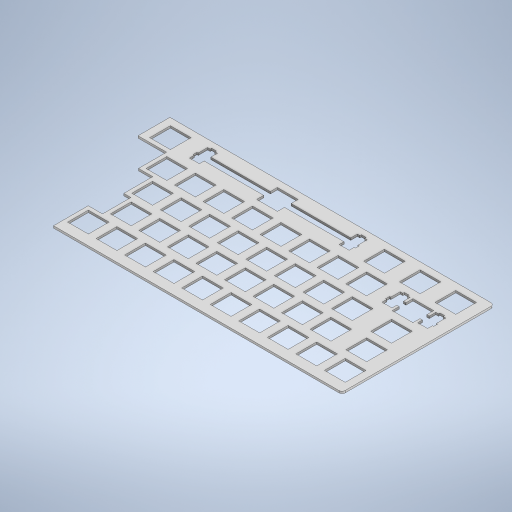
# Autodesk Inventor part: case_plate_p1
Saved by Autodesk Inventor 2024 (Build 280153000, 153)
## iProperties
Created: 2023-08-02
Part Number: case_plate_p1
Material: Generic
Document SubType Name: Modeling
Designer: Mika
Density: 1 g/cm^3
Appearance: Default
Author: Mika
Autodesk Inventor part; units mm, degrees
ref_plane "YZ Plane" through (0, 0, 0) normal (1, 0, 0) x (0, 1, 0)
ref_plane "XZ Plane" through (0, 0, 0) normal (0, 1, 0) x (-1, 0, 0)
ref_plane "XY Plane" through (0, 0, 0) normal (0, 0, 1) x (1, 0, 0)
sketch "Sketch1" plane through (0, 0, 0) normal (0, 1, 0) x (-1, 0, 0)
  line L0 (309.0479, 99.8402) -> (309.0479, 2.3404)
  line L1 (307.045, 0.3402) -> (2.0931, 0.3389)
  line L2 (0.096, 2.3404) -> (0.096, 99.8389)
  line L3 (2.096, 101.8389) -> (307.045, 101.8402)
  line L4 (126.213, 18.8654) -> (126.213, 14.1663)
  line L5 (126.213, 14.1663) -> (86.4387, 14.1663)
  line L6 (86.4387, 14.1663) -> (86.4387, 17.395)
  line L7 (86.4387, 17.395) -> (84.7136, 17.395)
  line L8 (81.5633, 17.395) -> (79.8382, 17.395)
  line L9 (79.8382, 17.395) -> (79.8382, 14.1663)
  line L10 (79.8382, 14.1663) -> (79.0141, 14.1663)
  line L11 (79.0141, 14.1663) -> (79.0141, 11.5163)
  line L12 (79.0141, 11.5163) -> (79.8382, 11.5163)
  line L13 (79.8382, 11.5163) -> (79.8382, 5.2462)
  line L14 (79.8382, 5.2462) -> (81.5633, 5.2462)
  line L15 (81.5633, 5.2462) -> (81.5633, 4.265)
  line L16 (81.5633, 4.265) -> (84.7136, 4.265)
  line L17 (84.7136, 4.265) -> (84.7136, 5.2462)
  line L18 (84.7136, 5.2462) -> (86.4387, 5.2462)
  line L19 (86.4387, 5.2462) -> (86.4387, 9.7166)
  line L20 (86.4387, 9.7166) -> (126.213, 9.7166)
  line L21 (126.213, 9.7166) -> (126.213, 5.0161)
  line L22 (126.213, 5.0161) -> (140.064, 5.0161)
  line L23 (140.064, 5.0161) -> (140.064, 9.7166)
  line L24 (140.064, 9.7166) -> (179.838, 9.7166)
  line L25 (179.838, 9.7166) -> (179.838, 5.2462)
  line L26 (179.838, 5.2462) -> (181.563, 5.2462)
  line L27 (181.563, 5.2462) -> (181.563, 4.265)
  line L28 (181.563, 4.265) -> (184.714, 4.265)
  line L29 (184.714, 4.265) -> (184.714, 5.2462)
  line L30 (184.714, 5.2462) -> (186.439, 5.2462)
  line L31 (186.439, 5.2462) -> (186.439, 11.5163)
  line L32 (186.439, 11.5163) -> (187.263, 11.5163)
  line L33 (187.263, 11.5163) -> (187.263, 14.1663)
  line L34 (187.263, 14.1663) -> (186.439, 14.1663)
  line L35 (186.439, 14.1663) -> (186.439, 17.395)
  line L36 (186.439, 17.395) -> (184.714, 17.395)
  line L37 (181.563, 17.395) -> (179.838, 17.395)
  line L38 (179.838, 17.395) -> (179.838, 14.1663)
  line L39 (179.838, 14.1663) -> (140.064, 14.1663)
  line L40 (140.064, 14.1663) -> (140.064, 18.8654)
  line L41 (140.064, 18.8654) -> (126.213, 18.8654)
  line L42 (7.152, 18.8654) -> (21.0013, 18.8654)
  line L43 (21.0013, 18.8654) -> (21.0013, 5.0161)
  line L44 (21.0013, 5.0161) -> (7.152, 5.0161)
  line L45 (7.152, 5.0161) -> (7.152, 18.8654)
  line L46 (30.9631, 18.8654) -> (44.8137, 18.8654)
  line L47 (44.8137, 18.8654) -> (44.8137, 5.0161)
  line L48 (44.8137, 5.0161) -> (30.9631, 5.0161)
  line L49 (30.9631, 5.0161) -> (30.9631, 18.8654)
  line L50 (54.7769, 18.8654) -> (68.6262, 18.8654)
  line L51 (68.6262, 18.8654) -> (68.6262, 5.0161)
  line L52 (68.6262, 5.0161) -> (54.7769, 5.0161)
  line L53 (54.7769, 5.0161) -> (54.7769, 18.8654)
  line L54 (197.652, 18.8654) -> (211.501, 18.8654)
  line L55 (211.501, 18.8654) -> (211.501, 5.0161)
  line L56 (211.501, 5.0161) -> (197.652, 5.0161)
  line L57 (197.652, 5.0161) -> (197.652, 18.8654)
  line L58 (221.463, 18.8654) -> (235.314, 18.8654)
  line L59 (235.314, 18.8654) -> (235.314, 5.0161)
  line L60 (235.314, 5.0161) -> (221.463, 5.0161)
  line L61 (221.463, 5.0161) -> (221.463, 18.8654)
  line L62 (252.421, 18.8654) -> (266.27, 18.8654)
  line L63 (266.27, 18.8654) -> (266.27, 5.0161)
  line L64 (266.27, 5.0161) -> (252.421, 5.0161)
  line L65 (252.421, 5.0161) -> (252.421, 18.8654)
  line L66 (271.471, 18.8654) -> (285.32, 18.8654)
  line L67 (285.32, 18.8654) -> (285.32, 5.0161)
  line L68 (285.32, 5.0161) -> (271.471, 5.0161)
  line L69 (271.471, 5.0161) -> (271.471, 18.8654)
  line L70 (290.521, 18.8654) -> (304.37, 18.8654)
  line L71 (304.37, 18.8654) -> (304.37, 5.0161)
  line L72 (304.37, 5.0161) -> (290.521, 5.0161)
  line L73 (290.521, 5.0161) -> (290.521, 18.8654)
  line L74 (16.677, 37.9155) -> (16.677, 33.2163)
  line L75 (16.677, 33.2163) -> (15.0013, 33.2163)
  line L76 (15.0013, 33.2163) -> (15.0013, 36.4451)
  line L77 (15.0013, 36.4451) -> (13.276, 36.4451)
  line L78 (10.1258, 36.4451) -> (8.4019, 36.4451)
  line L79 (8.4019, 36.4451) -> (8.4019, 33.2163)
  line L80 (8.4019, 33.2163) -> (7.5765, 33.2163)
  line L81 (7.5765, 33.2163) -> (7.5765, 30.5663)
  line L82 (7.5765, 30.5663) -> (8.4019, 30.5663)
  line L83 (8.4019, 30.5663) -> (8.4019, 24.2962)
  line L84 (8.4019, 24.2962) -> (10.1258, 24.2962)
  line L85 (10.1258, 24.2962) -> (10.1258, 23.315)
  line L86 (10.1258, 23.315) -> (13.276, 23.315)
  line L87 (13.276, 23.315) -> (13.276, 24.2962)
  line L88 (13.276, 24.2962) -> (15.0013, 24.2962)
  line L89 (15.0013, 24.2962) -> (15.0013, 28.7652)
  line L90 (15.0013, 28.7652) -> (16.677, 28.7652)
  line L91 (16.677, 28.7652) -> (16.677, 24.0661)
  line L92 (16.677, 24.0661) -> (30.5263, 24.0661)
  line L93 (30.5263, 24.0661) -> (30.5263, 28.7652)
  line L94 (30.5263, 28.7652) -> (32.202, 28.7652)
  line L95 (32.202, 28.7652) -> (32.202, 24.2962)
  line L96 (32.202, 24.2962) -> (33.9259, 24.2962)
  line L97 (33.9259, 24.2962) -> (33.9259, 23.315)
  line L98 (33.9259, 23.315) -> (37.0762, 23.315)
  line L99 (37.0762, 23.315) -> (37.0762, 24.2962)
  line L100 (37.0762, 24.2962) -> (38.8013, 24.2962)
  line L101 (38.8013, 24.2962) -> (38.8013, 30.5663)
  line L102 (38.8013, 30.5663) -> (39.6268, 30.5663)
  line L103 (39.6268, 30.5663) -> (39.6268, 33.2163)
  line L104 (39.6268, 33.2163) -> (38.8013, 33.2163)
  line L105 (38.8013, 33.2163) -> (38.8013, 36.4451)
  line L106 (38.8013, 36.4451) -> (37.0762, 36.4451)
  line L107 (33.9259, 36.4451) -> (32.202, 36.4451)
  line L108 (32.202, 36.4451) -> (32.202, 33.2163)
  line L109 (32.202, 33.2163) -> (30.5263, 33.2163)
  line L110 (30.5263, 33.2163) -> (30.5263, 37.9155)
  line L111 (30.5263, 37.9155) -> (16.677, 37.9155)
  line L112 (47.6321, 37.9155) -> (61.4825, 37.9155)
  line L113 (61.4825, 37.9155) -> (61.4825, 24.0661)
  line L114 (61.4825, 24.0661) -> (47.6321, 24.0661)
  line L115 (47.6321, 24.0661) -> (47.6321, 37.9155)
  line L116 (66.6821, 37.9155) -> (80.5325, 37.9155)
  line L117 (80.5325, 37.9155) -> (80.5325, 24.0661)
  line L118 (80.5325, 24.0661) -> (66.6821, 24.0661)
  line L119 (66.6821, 24.0661) -> (66.6821, 37.9155)
  line L120 (85.7321, 37.9155) -> (99.5825, 37.9155)
  line L121 (99.5825, 37.9155) -> (99.5825, 24.0661)
  line L122 (99.5825, 24.0661) -> (85.7321, 24.0661)
  line L123 (85.7321, 24.0661) -> (85.7321, 37.9155)
  line L124 (104.782, 37.9155) -> (118.632, 37.9155)
  line L125 (118.632, 37.9155) -> (118.632, 24.0661)
  line L126 (118.632, 24.0661) -> (104.782, 24.0661)
  line L127 (104.782, 24.0661) -> (104.782, 37.9155)
  line L128 (123.832, 37.9155) -> (137.682, 37.9155)
  line L129 (137.682, 37.9155) -> (137.682, 24.0661)
  line L130 (137.682, 24.0661) -> (123.832, 24.0661)
  line L131 (123.832, 24.0661) -> (123.832, 37.9155)
  line L132 (142.882, 37.9155) -> (156.732, 37.9155)
  line L133 (156.732, 37.9155) -> (156.732, 24.0661)
  line L134 (156.732, 24.0661) -> (142.882, 24.0661)
  line L135 (142.882, 24.0661) -> (142.882, 37.9155)
  line L136 (161.932, 37.9155) -> (175.782, 37.9155)
  line L137 (175.782, 37.9155) -> (175.782, 24.0661)
  line L138 (175.782, 24.0661) -> (161.932, 24.0661)
  line L139 (161.932, 24.0661) -> (161.932, 37.9155)
  line L140 (180.982, 37.9155) -> (194.832, 37.9155)
  line L141 (194.832, 37.9155) -> (194.832, 24.0661)
  line L142 (194.832, 24.0661) -> (180.982, 24.0661)
  line L143 (180.982, 24.0661) -> (180.982, 37.9155)
  line L144 (200.032, 37.9155) -> (213.882, 37.9155)
  line L145 (213.882, 37.9155) -> (213.882, 24.0661)
  line L146 (213.882, 24.0661) -> (200.032, 24.0661)
  line L147 (200.032, 24.0661) -> (200.032, 37.9155)
  line L148 (219.082, 37.9155) -> (232.932, 37.9155)
  line L149 (232.932, 37.9155) -> (232.932, 24.0661)
  line L150 (232.932, 24.0661) -> (219.082, 24.0661)
  line L151 (219.082, 24.0661) -> (219.082, 37.9155)
  line L152 (245.277, 37.9155) -> (259.126, 37.9155)
  line L153 (259.126, 37.9155) -> (259.126, 24.0661)
  line L154 (259.126, 24.0661) -> (245.277, 24.0661)
  line L155 (245.277, 24.0661) -> (245.277, 37.9155)
  line L156 (271.471, 37.9155) -> (285.32, 37.9155)
  line L157 (285.32, 37.9155) -> (285.32, 24.0661)
  line L158 (285.32, 24.0661) -> (271.471, 24.0661)
  line L159 (271.471, 24.0661) -> (271.471, 37.9155)
  line L160 (290.521, 37.9155) -> (304.37, 37.9155)
  line L161 (304.37, 37.9155) -> (304.37, 24.0661)
  line L162 (304.37, 24.0661) -> (290.521, 24.0661)
  line L163 (290.521, 24.0661) -> (290.521, 37.9155)
  line L164 (259.563, 56.9655) -> (259.563, 52.2661)
  line L165 (259.563, 52.2661) -> (257.889, 52.2661)
  line L166 (257.889, 52.2661) -> (257.889, 55.4951)
  line L167 (257.889, 55.4951) -> (256.162, 55.4951)
  line L168 (253.013, 55.4951) -> (251.288, 55.4951)
  line L169 (251.288, 55.4951) -> (251.288, 52.2661)
  line L170 (251.288, 52.2661) -> (250.464, 52.2661)
  line L171 (250.464, 52.2661) -> (250.464, 49.6164)
  line L172 (250.464, 49.6164) -> (251.288, 49.6164)
  line L173 (251.288, 49.6164) -> (251.288, 43.3462)
  line L174 (251.288, 43.3462) -> (253.013, 43.3462)
  line L175 (253.013, 43.3462) -> (253.013, 42.3651)
  line L176 (253.013, 42.3651) -> (256.162, 42.3651)
  line L177 (256.162, 42.3651) -> (256.162, 43.3462)
  line L178 (256.162, 43.3462) -> (257.889, 43.3462)
  line L179 (257.889, 43.3462) -> (257.889, 47.8151)
  line L180 (257.889, 47.8151) -> (259.563, 47.8151)
  line L181 (259.563, 47.8151) -> (259.563, 43.1161)
  line L182 (259.563, 43.1161) -> (273.414, 43.1161)
  line L183 (273.414, 43.1161) -> (273.414, 47.8151)
  line L184 (273.414, 47.8151) -> (275.088, 47.8151)
  line L185 (275.088, 47.8151) -> (275.088, 43.3462)
  line L186 (275.088, 43.3462) -> (276.813, 43.3462)
  line L187 (276.813, 43.3462) -> (276.813, 42.3651)
  line L188 (276.813, 42.3651) -> (279.964, 42.3651)
  line L189 (279.964, 42.3651) -> (279.964, 43.3462)
  line L190 (279.964, 43.3462) -> (281.689, 43.3462)
  line L191 (281.689, 43.3462) -> (281.689, 49.6164)
  line L192 (281.689, 49.6164) -> (282.513, 49.6164)
  line L193 (282.513, 49.6164) -> (282.513, 52.2661)
  line L194 (282.513, 52.2661) -> (281.689, 52.2661)
  line L195 (281.689, 52.2661) -> (281.689, 55.4951)
  line L196 (281.689, 55.4951) -> (279.964, 55.4951)
  line L197 (276.813, 55.4951) -> (275.088, 55.4951)
  line L198 (275.088, 55.4951) -> (275.088, 52.2661)
  line L199 (275.088, 52.2661) -> (273.414, 52.2661)
  line L200 (273.414, 52.2661) -> (273.414, 56.9655)
  line L201 (273.414, 56.9655) -> (259.563, 56.9655)
  line L202 (11.9131, 56.9655) -> (25.7638, 56.9655)
  line L203 (25.7638, 56.9655) -> (25.7638, 43.1161)
  line L204 (25.7638, 43.1161) -> (11.9131, 43.1161)
  line L205 (11.9131, 43.1161) -> (11.9131, 56.9655)
  line L206 (38.1071, 56.9655) -> (51.9575, 56.9655)
  line L207 (51.9575, 56.9655) -> (51.9575, 43.1161)
  line L208 (51.9575, 43.1161) -> (38.1071, 43.1161)
  line L209 (38.1071, 43.1161) -> (38.1071, 56.9655)
  line L210 (57.1571, 56.9655) -> (71.0075, 56.9655)
  line L211 (71.0075, 56.9655) -> (71.0075, 43.1161)
  line L212 (71.0075, 43.1161) -> (57.1571, 43.1161)
  line L213 (57.1571, 43.1161) -> (57.1571, 56.9655)
  line L214 (76.2071, 56.9655) -> (90.0575, 56.9655)
  line L215 (90.0575, 56.9655) -> (90.0575, 43.1161)
  line L216 (90.0575, 43.1161) -> (76.2071, 43.1161)
  line L217 (76.2071, 43.1161) -> (76.2071, 56.9655)
  line L218 (95.2571, 56.9655) -> (109.107, 56.9655)
  line L219 (109.107, 56.9655) -> (109.107, 43.1161)
  line L220 (109.107, 43.1161) -> (95.2571, 43.1161)
  line L221 (95.2571, 43.1161) -> (95.2571, 56.9655)
  line L222 (114.307, 56.9655) -> (128.157, 56.9655)
  line L223 (128.157, 56.9655) -> (128.157, 43.1161)
  line L224 (128.157, 43.1161) -> (114.307, 43.1161)
  line L225 (114.307, 43.1161) -> (114.307, 56.9655)
  line L226 (133.357, 56.9655) -> (147.207, 56.9655)
  line L227 (147.207, 56.9655) -> (147.207, 43.1161)
  line L228 (147.207, 43.1161) -> (133.357, 43.1161)
  line L229 (133.357, 43.1161) -> (133.357, 56.9655)
  line L230 (152.407, 56.9655) -> (166.257, 56.9655)
  line L231 (166.257, 56.9655) -> (166.257, 43.1161)
  line L232 (166.257, 43.1161) -> (152.407, 43.1161)
  line L233 (152.407, 43.1161) -> (152.407, 56.9655)
  line L234 (171.457, 56.9655) -> (185.307, 56.9655)
  line L235 (185.307, 56.9655) -> (185.307, 43.1161)
  line L236 (185.307, 43.1161) -> (171.457, 43.1161)
  line L237 (171.457, 43.1161) -> (171.457, 56.9655)
  line L238 (190.507, 56.9655) -> (204.357, 56.9655)
  line L239 (204.357, 56.9655) -> (204.357, 43.1161)
  line L240 (204.357, 43.1161) -> (190.507, 43.1161)
  line L241 (190.507, 43.1161) -> (190.507, 56.9655)
  line L242 (209.557, 56.9655) -> (223.407, 56.9655)
  line L243 (223.407, 56.9655) -> (223.407, 43.1161)
  line L244 (223.407, 43.1161) -> (209.557, 43.1161)
  line L245 (209.557, 43.1161) -> (209.557, 56.9655)
  line L246 (228.607, 56.9655) -> (242.457, 56.9655)
  line L247 (242.457, 56.9655) -> (242.457, 43.1161)
  line L248 (242.457, 43.1161) -> (228.607, 43.1161)
  line L249 (228.607, 43.1161) -> (228.607, 56.9655)
  line L250 (290.521, 56.9655) -> (304.37, 56.9655)
  line L251 (304.37, 56.9655) -> (304.37, 43.1161)
  line L252 (304.37, 43.1161) -> (290.521, 43.1161)
  line L253 (290.521, 43.1161) -> (290.521, 56.9655)
  line L254 (9.5319, 76.0155) -> (23.3826, 76.0155)
  line L255 (23.3826, 76.0155) -> (23.3826, 62.1661)
  line L256 (23.3826, 62.1661) -> (9.5319, 62.1661)
  line L257 (9.5319, 62.1661) -> (9.5319, 76.0155)
  line L258 (33.3458, 76.0155) -> (47.195, 76.0155)
  line L259 (47.195, 76.0155) -> (47.195, 62.1661)
  line L260 (47.195, 62.1661) -> (33.3458, 62.1661)
  line L261 (33.3458, 62.1661) -> (33.3458, 76.0155)
  line L262 (52.3956, 76.0155) -> (66.245, 76.0155)
  line L263 (66.245, 76.0155) -> (66.245, 62.1661)
  line L264 (66.245, 62.1661) -> (52.3956, 62.1661)
  line L265 (52.3956, 62.1661) -> (52.3956, 76.0155)
  line L266 (71.4456, 76.0155) -> (85.295, 76.0155)
  line L267 (85.295, 76.0155) -> (85.295, 62.1661)
  line L268 (85.295, 62.1661) -> (71.4456, 62.1661)
  line L269 (71.4456, 62.1661) -> (71.4456, 76.0155)
  line L270 (90.4946, 76.0155) -> (104.345, 76.0155)
  line L271 (104.345, 76.0155) -> (104.345, 62.1661)
  line L272 (104.345, 62.1661) -> (90.4946, 62.1661)
  line L273 (90.4946, 62.1661) -> (90.4946, 76.0155)
  line L274 (109.545, 76.0155) -> (123.395, 76.0155)
  line L275 (123.395, 76.0155) -> (123.395, 62.1661)
  line L276 (123.395, 62.1661) -> (109.545, 62.1661)
  line L277 (109.545, 62.1661) -> (109.545, 76.0155)
  line L278 (128.595, 76.0155) -> (142.445, 76.0155)
  line L279 (142.445, 76.0155) -> (142.445, 62.1661)
  line L280 (142.445, 62.1661) -> (128.595, 62.1661)
  line L281 (128.595, 62.1661) -> (128.595, 76.0155)
  line L282 (147.645, 76.0155) -> (161.495, 76.0155)
  line L283 (161.495, 76.0155) -> (161.495, 62.1661)
  line L284 (161.495, 62.1661) -> (147.645, 62.1661)
  line L285 (147.645, 62.1661) -> (147.645, 76.0155)
  line L286 (166.696, 76.0155) -> (180.545, 76.0155)
  line L287 (180.545, 76.0155) -> (180.545, 62.1661)
  line L288 (180.545, 62.1661) -> (166.696, 62.1661)
  line L289 (166.696, 62.1661) -> (166.696, 76.0155)
  line L290 (185.746, 76.0155) -> (199.595, 76.0155)
  line L291 (199.595, 76.0155) -> (199.595, 62.1661)
  line L292 (199.595, 62.1661) -> (185.746, 62.1661)
  line L293 (185.746, 62.1661) -> (185.746, 76.0155)
  line L294 (204.796, 76.0155) -> (218.645, 76.0155)
  line L295 (218.645, 76.0155) -> (218.645, 62.1661)
  line L296 (218.645, 62.1661) -> (204.796, 62.1661)
  line L297 (204.796, 62.1661) -> (204.796, 76.0155)
  line L298 (223.846, 76.0155) -> (237.695, 76.0155)
  line L299 (237.695, 76.0155) -> (237.695, 62.1661)
  line L300 (237.695, 62.1661) -> (223.846, 62.1661)
  line L301 (223.846, 62.1661) -> (223.846, 76.0155)
  line L302 (242.896, 76.0155) -> (256.745, 76.0155)
  line L303 (256.745, 76.0155) -> (256.745, 62.1661)
  line L304 (256.745, 62.1661) -> (242.896, 62.1661)
  line L305 (242.896, 62.1661) -> (242.896, 76.0155)
  line L306 (266.707, 76.0155) -> (280.557, 76.0155)
  line L307 (280.557, 76.0155) -> (280.557, 62.1661)
  line L308 (280.557, 62.1661) -> (266.707, 62.1661)
  line L309 (266.707, 62.1661) -> (266.707, 76.0155)
  line L310 (290.521, 76.0155) -> (304.37, 76.0155)
  line L311 (304.37, 76.0155) -> (304.37, 62.1661)
  line L312 (304.37, 62.1661) -> (290.521, 62.1661)
  line L313 (290.521, 62.1661) -> (290.521, 76.0155)
  line L314 (261.946, 95.0655) -> (261.946, 90.3661)
  line L315 (261.946, 90.3661) -> (260.27, 90.3661)
  line L316 (260.27, 90.3661) -> (260.27, 93.5951)
  line L317 (260.27, 93.5951) -> (258.546, 93.5951)
  line L318 (255.396, 93.5951) -> (253.67, 93.5951)
  line L319 (253.67, 93.5951) -> (253.67, 90.3661)
  line L320 (253.67, 90.3661) -> (252.845, 90.3661)
  line L321 (252.845, 90.3661) -> (252.845, 87.7164)
  line L322 (252.845, 87.7164) -> (253.67, 87.7164)
  line L323 (253.67, 87.7164) -> (253.67, 81.4462)
  line L324 (253.67, 81.4462) -> (255.396, 81.4462)
  line L325 (255.396, 81.4462) -> (255.396, 80.4651)
  line L326 (255.396, 80.4651) -> (258.546, 80.4651)
  line L327 (258.546, 80.4651) -> (258.546, 81.4462)
  line L328 (258.546, 81.4462) -> (260.27, 81.4462)
  line L329 (260.27, 81.4462) -> (260.27, 85.9151)
  line L330 (260.27, 85.9151) -> (261.946, 85.9151)
  line L331 (261.946, 85.9151) -> (261.946, 81.2161)
  line L332 (261.946, 81.2161) -> (275.795, 81.2161)
  line L333 (275.795, 81.2161) -> (275.795, 85.9151)
  line L334 (275.795, 85.9151) -> (277.471, 85.9151)
  line L335 (277.471, 85.9151) -> (277.471, 81.4462)
  line L336 (277.471, 81.4462) -> (279.196, 81.4462)
  line L337 (279.196, 81.4462) -> (279.196, 80.4651)
  line L338 (279.196, 80.4651) -> (282.345, 80.4651)
  line L339 (282.345, 80.4651) -> (282.345, 81.4462)
  line L340 (282.345, 81.4462) -> (284.07, 81.4462)
  line L341 (284.07, 81.4462) -> (284.07, 87.7164)
  line L342 (284.07, 87.7164) -> (284.896, 87.7164)
  line L343 (284.896, 87.7164) -> (284.896, 90.3661)
  line L344 (284.896, 90.3661) -> (284.07, 90.3661)
  line L345 (284.07, 90.3661) -> (284.07, 93.5951)
  line L346 (284.07, 93.5951) -> (282.345, 93.5951)
  line L347 (279.196, 93.5951) -> (277.471, 93.5951)
  line L348 (277.471, 93.5951) -> (277.471, 90.3661)
  line L349 (277.471, 90.3661) -> (275.795, 90.3661)
  line L350 (275.795, 90.3661) -> (275.795, 95.0655)
  line L351 (275.795, 95.0655) -> (261.946, 95.0655)
  line L352 (4.7708, 95.0655) -> (18.6201, 95.0655)
  line L353 (18.6201, 95.0655) -> (18.6201, 81.2161)
  line L354 (18.6201, 81.2161) -> (4.7708, 81.2161)
  line L355 (4.7708, 81.2161) -> (4.7708, 95.0655)
  line L356 (23.8208, 95.0655) -> (37.67, 95.0655)
  line L357 (37.67, 95.0655) -> (37.67, 81.2161)
  line L358 (37.67, 81.2161) -> (23.8208, 81.2161)
  line L359 (23.8208, 81.2161) -> (23.8208, 95.0655)
  line L360 (42.8706, 95.0655) -> (56.72, 95.0655)
  line L361 (56.72, 95.0655) -> (56.72, 81.2161)
  line L362 (56.72, 81.2161) -> (42.8706, 81.2161)
  line L363 (42.8706, 81.2161) -> (42.8706, 95.0655)
  line L364 (61.9206, 95.0655) -> (75.77, 95.0655)
  line L365 (75.77, 95.0655) -> (75.77, 81.2161)
  line L366 (75.77, 81.2161) -> (61.9206, 81.2161)
  line L367 (61.9206, 81.2161) -> (61.9206, 95.0655)
  line L368 (80.9706, 95.0655) -> (94.82, 95.0655)
  line L369 (94.82, 95.0655) -> (94.82, 81.2161)
  line L370 (94.82, 81.2161) -> (80.9706, 81.2161)
  line L371 (80.9706, 81.2161) -> (80.9706, 95.0655)
  line L372 (100.021, 95.0655) -> (113.87, 95.0655)
  line L373 (113.87, 95.0655) -> (113.87, 81.2161)
  line L374 (113.87, 81.2161) -> (100.021, 81.2161)
  line L375 (100.021, 81.2161) -> (100.021, 95.0655)
  line L376 (119.071, 95.0655) -> (132.92, 95.0655)
  line L377 (132.92, 95.0655) -> (132.92, 81.2161)
  line L378 (132.92, 81.2161) -> (119.071, 81.2161)
  line L379 (119.071, 81.2161) -> (119.071, 95.0655)
  line L380 (138.121, 95.0655) -> (151.97, 95.0655)
  line L381 (151.97, 95.0655) -> (151.97, 81.2161)
  line L382 (151.97, 81.2161) -> (138.121, 81.2161)
  line L383 (138.121, 81.2161) -> (138.121, 95.0655)
  line L384 (157.171, 95.0655) -> (171.02, 95.0655)
  line L385 (171.02, 95.0655) -> (171.02, 81.2161)
  line L386 (171.02, 81.2161) -> (157.171, 81.2161)
  line L387 (157.171, 81.2161) -> (157.171, 95.0655)
  line L388 (176.221, 95.0655) -> (190.07, 95.0655)
  line L389 (190.07, 95.0655) -> (190.07, 81.2161)
  line L390 (190.07, 81.2161) -> (176.221, 81.2161)
  line L391 (176.221, 81.2161) -> (176.221, 95.0655)
  line L392 (195.271, 95.0655) -> (209.12, 95.0655)
  line L393 (209.12, 95.0655) -> (209.12, 81.2161)
  line L394 (209.12, 81.2161) -> (195.271, 81.2161)
  line L395 (195.271, 81.2161) -> (195.271, 95.0655)
  line L396 (214.321, 95.0655) -> (228.17, 95.0655)
  line L397 (228.17, 95.0655) -> (228.17, 81.2161)
  line L398 (228.17, 81.2161) -> (214.321, 81.2161)
  line L399 (214.321, 81.2161) -> (214.321, 95.0655)
  line L400 (233.371, 95.0655) -> (247.22, 95.0655)
  line L401 (247.22, 95.0655) -> (247.22, 81.2161)
  line L402 (247.22, 81.2161) -> (233.371, 81.2161)
  line L403 (233.371, 81.2161) -> (233.371, 95.0655)
  line L404 (290.521, 95.0655) -> (304.37, 95.0655)
  line L405 (304.37, 95.0655) -> (304.37, 81.2161)
  line L406 (304.37, 81.2161) -> (290.521, 81.2161)
  line L407 (290.521, 81.2161) -> (290.521, 95.0655)
  arc A0 (307.045, 0.3402) -> (309.0479, 2.3404) centre (307.0479, 2.3402) ccw
  arc A1 (0.096, 2.3404) -> (2.0931, 0.3389) centre (2.096, 2.3389) ccw
  arc A2 (309.0479, 99.8402) -> (307.045, 101.8402) centre (307.0479, 99.8402) ccw
  arc A3 (2.096, 101.8389) -> (0.096, 99.8389) centre (2.096, 99.8389) ccw
  line L408 (221.0479, 101.8399) -> (221.0479, 99.8399)
  line L409 (221.0479, 99.8399) -> (236.0479, 99.8399)
  line L410 (221.0479, 99.8399) -> (206.0479, 99.8399)
  line L411 (221.0479, 99.8399) -> (236.0479, 99.8399) construction
  circle A4 centre (221.0479, 99.8399) radius 1.75
  circle A5 centre (206.0479, 99.8399) radius 1.75
  circle A6 centre (236.0479, 99.8399) radius 1.75
  line L412 (187.907, 40.376) -> (187.907, 59.7445)
  line L413 (187.907, 59.7445) -> (183.1445, 59.7445)
  line L414 (183.1445, 59.7445) -> (183.1445, 78.7061)
  line L415 (183.1445, 78.7061) -> (192.6705, 78.7061)
  line L416 (192.6705, 78.7061) -> (192.6704, 101.8397)
  line L417 (187.907, 40.376) -> (197.432, 40.376)
  line L418 (197.432, 40.376) -> (197.432, 21.6053)
  line L419 (197.432, 21.6053) -> (216.482, 21.6053)
  line L420 (216.482, 21.6053) -> (216.4821, 0.3398)
  line L421 (10.1258, 36.4451) -> (13.276, 36.4451)
  line L422 (33.9259, 36.4451) -> (37.0762, 36.4451)
  line L423 (81.5633, 17.395) -> (84.7136, 17.395)
  line L424 (181.563, 17.395) -> (184.714, 17.395)
  line L425 (253.013, 55.4951) -> (256.162, 55.4951)
  line L426 (276.813, 55.4951) -> (279.964, 55.4951)
  line L427 (282.345, 93.5951) -> (279.196, 93.5951)
  line L428 (258.546, 93.5951) -> (255.396, 93.5951)
  point P0 (4.7708, 81.2161)
  point P1 (7.152, 5.0161)
  point P2 (193.4145, 0.3397)
  dimension "d0" = 308.9519
  dimension "d1" = 101.5
  dimension "d12" = 88
  dimension "d13" = 2
  dimension "d14" = 15
  dimension "d15" = 15
  dimension "d16" = 180
  dimension "d20" = 3.5
  dimension "d21" = 3.5
  dimension "d22" = 3.5
  constraints: 864 end point, 8 point on circle, 7 centre point, 7 horizontal, 6 perpendicular, 5 collinear, 4 coincident, 4 point on line, 3 parallel, 1 vertical
  measures "d0" distance between parallel lines of L0 L2
  measures "d1" distance between parallel lines of L3 L1
  measures "d12" distance from line of L0.start L408
  measures "d13" distance of L408.start L408.end
  measures "d14" distance of L409.start L409.end
  measures "d15" distance of L409.start L410.end
  measures "d16" angle of L410 L411
  measures "d20" diameter of A4
  measures "d21" diameter of A5
  measures "d22" diameter of A6
extrude "Extrusion4" add sketch "Sketch1" along normal blind 1.4 contours L1 A1 L2 A3 L3 L416 L415 L414 L413 L412 L417 L418 L419 L420
body "Solid3"
